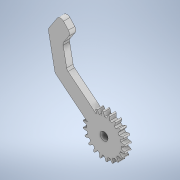
# Autodesk Inventor part: Servo pinza 1
Saved by Autodesk Inventor 2021 (Build 250183000, 183)
## iProperties
Created: 2021-03-25
Part Number: Servo pinza 1
Material: Generic
Document SubType Name: Modeling
Designer: LCG
Density: 1 g/cm^3
Appearance: Default
Author: LCG
Autodesk Inventor part; units mm, degrees
ref_plane "YZ Plane" through (0, 0, 0) normal (1, 0, 0) x (0, 1, 0)
ref_plane "XZ Plane" through (0, 0, 0) normal (0, 1, 0) x (-1, 0, 0)
ref_plane "XY Plane" through (0, 0, 0) normal (0, 0, 1) x (1, 0, 0)
sketch "Sketch1" plane through (0, 0, 0) normal (0, 0, 1) x (1, 0, 0)
  circle A0 centre (0, 0) radius 2.5
  line L0 (0, 0) -> (-15.5714, 12.5511)
  line L1 (0, 0) -> (20, 0) construction
  line L2 (-15.5714, 12.5511) -> (-18.3421, 9.1137)
  line L3 (0, 0) -> (-10.3273, 2.6535)
  line L4 (0, 0) -> (22.7557, 0) construction
  line L5 (0, 0) -> (-10.6628, 0)
  line L6 (-4.786, 9.5283) -> (-22.3661, 23.6985)
  line L7 (-22.3661, 23.6985) -> (-20.7973, 25.6449)
  circle A1 centre (-20.7973, 25.6449) radius 2.5
  line L8 (-18.3421, 9.1137) -> (-10.3273, 2.6535)
  line L9 (-23.2502, 25.1624) -> (-25.4393, 36.2891)
  line L10 (-23.2502, 25.1624) -> (-11.9102, 25.1624) construction
  line L11 (-25.4393, 36.2891) -> (-22.9863, 36.7717)
  circle A2 centre (-22.9863, 36.7717) radius 2.5
  line L12 (-25.0727, 38.149) -> (-21.9049, 42.9477)
  line L13 (-25.0727, 38.149) -> (-19.3227, 38.149) construction
  line L14 (-21.9049, 42.9477) -> (-23.9913, 44.325)
  circle A3 centre (-23.9913, 44.325) radius 2.5
  line L15 (0, 0) -> (60, 0) construction
  line L16 (-25.2189, 49.3225) -> (-22.1589, 46.0257)
  line L17 (-23.9913, 39.7871) -> (-31.8111, 44.9492)
  line L18 (-31.8111, 44.9492) -> (-29.1376, 48.9991)
  line L19 (-31.8111, 44.9492) -> (-34.1674, 41.3798)
  line L20 (-24.1412, 29.6912) -> (-32.2851, 28.089)
  line L21 (-32.2851, 28.089) -> (-34.534, 39.5199)
  line L22 (-32.2851, 28.089) -> (-30.6518, 19.787)
  line L23 (-18.3421, 9.1137) -> (-29.7677, 18.3232)
  line L24 (-18.3421, 20.455) -> (-23.8834, 13.5802)
  arc A4 (-12.5406, 2.5003) -> (-12.6967, 1.5208) centre (-12.5054, 1.9925) ccw
  line L25 (-10.3273, 2.6535) -> (-12.5406, 2.5003)
  line L26 (-10.6406, 0.6873) -> (-12.6967, 1.5208)
  line L27 (-10.6455, -0.6061) -> (-12.7079, -1.4239)
  line L28 (-10.3473, -2.5746) -> (-12.5593, -2.4045)
  arc A5 (-12.7079, -1.4239) -> (-12.5593, -2.4045) centre (-12.5203, -1.897) ccw
  line L29 (-9.9594, -3.8085) -> (-11.6763, -5.2137)
  line L30 (-9.0777, -5.5937) -> (-11.2371, -6.103)
  arc A6 (-11.6763, -5.2137) -> (-11.2371, -6.103) centre (-11.3539, -5.6076) ccw
  line L31 (-8.3337, -6.6517) -> (-9.5431, -8.5116)
  line L32 (-6.9518, -8.085) -> (-8.8547, -9.2257)
  arc A7 (-9.5431, -8.5116) -> (-8.8547, -9.2257) centre (-9.1164, -8.7891) ccw
  line L33 (-5.9217, -8.8672) -> (-6.5096, -11.0065)
  line L34 (-4.17, -9.8136) -> (-5.6369, -11.478)
  arc A8 (-6.5096, -11.0065) -> (-5.6369, -11.478) centre (-6.0188, -11.1414) ccw
  line L35 (-2.951, -10.2463) -> (-2.8619, -12.4631)
  line L36 (-0.9947, -10.6163) -> (-1.8873, -12.6474)
  arc A9 (-2.8619, -12.4631) -> (-1.8873, -12.6474) centre (-2.3533, -12.4426) ccw
  line L37 (0.298, -10.6586) -> (1.0558, -12.7438)
  line L38 (2.2743, -10.4174) -> (2.0403, -12.6236)
  arc A10 (1.0558, -12.7438) -> (2.0403, -12.6236) centre (1.5342, -12.5699) ccw
  line L39 (3.5189, -10.0654) -> (4.8738, -11.8222)
  line L40 (5.3288, -9.2357) -> (5.7755, -11.4089)
  arc A11 (4.8738, -11.8222) -> (5.7755, -11.4089) centre (5.2769, -11.5113) ccw
  line L41 (6.4079, -8.5225) -> (8.2321, -9.7852)
  line L42 (7.8806, -7.1827) -> (8.9658, -9.1178)
  arc A12 (8.2321, -9.7852) -> (8.9658, -9.1178) centre (8.5218, -9.3667) ccw
  line L43 (8.6923, -6.1756) -> (10.8137, -6.8251)
  line L44 (9.6889, -4.452) -> (11.3102, -5.9665)
  arc A13 (10.8137, -6.8251) -> (11.3102, -5.9665) centre (10.9627, -6.3384) ccw
  line L45 (10.1566, -3.2461) -> (12.3751, -3.2211)
  line L46 (10.5831, -1.3013) -> (12.5875, -2.2522)
  arc A14 (12.3751, -3.2211) -> (12.5875, -2.2522) centre (12.3693, -2.7121) ccw
  line L47 (10.6628, -0.0103) -> (12.769, 0.6868)
  line L48 (10.4788, 1.9721) -> (12.6773, 1.6744)
  arc A15 (12.769, 0.6868) -> (12.6773, 1.6744) centre (12.609, 1.17) ccw
  line L49 (10.1629, 3.2264) -> (11.9582, 4.5299)
  line L50 (9.3859, 5.0595) -> (11.5711, 5.4432)
  arc A16 (11.9582, 4.5299) -> (11.5711, 5.4432) centre (11.6591, 4.9418) ccw
  line L51 (8.7043, 6.1588) -> (10.0192, 7.9457)
  line L52 (7.4075, 7.6696) -> (9.3732, 8.6983)
  arc A17 (10.0192, 7.9457) -> (9.3732, 8.6983) centre (9.6092, 8.2474) ccw
  line L53 (6.4244, 8.5101) -> (7.135, 10.6118)
  line L54 (4.7303, 9.5561) -> (6.291, 11.1329)
  arc A18 (7.135, 10.6118) -> (6.291, 11.1329) centre (6.6528, 10.7748) ccw
  line L55 (3.5385, 10.0585) -> (3.5776, 12.2768)
  line L56 (1.6068, 10.541) -> (2.6153, 12.5171)
  arc A19 (3.5776, 12.2768) -> (2.6153, 12.5171) centre (3.0687, 12.2857) ccw
  line L57 (0.3187, 10.658) -> (-0.3173, 12.7835)
  line L58 (-1.6683, 10.5314) -> (-1.3071, 12.7204)
  arc A20 (-0.3173, 12.7835) -> (-1.3071, 12.7204) centre (-0.8049, 12.6376) ccw
  line L59 (-2.9312, 10.252) -> (-4.1823, 12.0842)
  line L60 (-4.786, 9.5283) -> (-5.1063, 11.7237)
  arc A21 (-4.1823, 12.0842) -> (-5.1063, 11.7237) centre (-4.6026, 11.7971) ccw
  arc A22 (-1.6683, 10.5314) -> (-2.9312, 10.252) centre (0, 0) ccw
  arc A23 (1.6068, 10.541) -> (0.3187, 10.658) centre (0, 0) ccw
  arc A24 (4.7303, 9.5561) -> (3.5385, 10.0585) centre (0, 0) ccw
  arc A25 (7.4075, 7.6696) -> (6.4244, 8.5101) centre (0, 0) ccw
  arc A26 (9.3859, 5.0595) -> (8.7043, 6.1588) centre (0, 0) ccw
  arc A27 (10.4788, 1.9721) -> (10.1629, 3.2264) centre (0, 0) ccw
  arc A28 (10.5831, -1.3013) -> (10.6628, 0) centre (0, 0) ccw
  arc A29 (9.6889, -4.452) -> (10.1566, -3.2461) centre (0, 0) ccw
  arc A30 (7.8806, -7.1827) -> (8.6923, -6.1756) centre (0, 0) ccw
  arc A31 (5.3288, -9.2357) -> (6.4079, -8.5225) centre (0, 0) ccw
  arc A32 (2.2743, -10.4174) -> (3.5189, -10.0654) centre (0, 0) ccw
  arc A33 (-0.9947, -10.6163) -> (0.298, -10.6586) centre (0, 0) ccw
  arc A34 (-4.17, -9.8136) -> (-2.951, -10.2463) centre (0, 0) ccw
  arc A35 (-6.9518, -8.085) -> (-5.9217, -8.8672) centre (0, 0) ccw
  arc A36 (-9.0777, -5.5937) -> (-8.3337, -6.6517) centre (0, 0) ccw
  arc A37 (-10.3473, -2.5746) -> (-9.9594, -3.8085) centre (0, 0) ccw
  arc A38 (-10.2331, 2.9964) -> (-10.3273, 2.6535) centre (0, 0) ccw
  arc A39 (-10.6406, 0.6873) -> (-10.6455, -0.6061) centre (0, 0) ccw
  line L61 (-4.9971, 9.2664) -> (-4.786, 9.5283)
  arc A40 (-25.2189, 49.3225) -> (-29.1376, 48.9991) centre (-27.0512, 47.6218) ccw
  arc A41 (-34.1674, 41.3798) -> (-34.534, 39.5199) centre (-32.081, 40.0025) ccw
  arc A42 (-30.6518, 19.787) -> (-29.7677, 18.3232) centre (-28.1988, 20.2696) ccw
  point P0 (-4.786, 9.5283)
  dimension "d0" = 5
  dimension "d1" = 20
  dimension "d2" = 141.13
  dimension "d3" = 4.415
  dimension "d4" = 165.59
  dimension "d5" = 22.58
  dimension "d6" = 2.5
  dimension "d10" = 11.34
  dimension "d12" = 101.13
  dimension "d13" = 2.5
  dimension "d15" = 5.75
  dimension "d17" = 56.57
  dimension "d18" = 2.5
  dimension "d22" = 9.37
  dimension "d23" = 8.3
  dimension "d24" = 8.83
  dimension "d25" = 1.991
  dimension "d27" = 1.018
  dimension "d30" = 300.366
  dimension "d32" = 2.5
  constraints: 124 end point, 85 point on circle, 43 centre point, 23 point on line, 15 perpendicular, 11 tangent, 6 horizontal, 5 coincident, 3 equal length, 2 equal radius, 137 other
  measures "d0" diameter of A0
  measures "d1" distance of L0.start L0.end
  measures "d2" angle of L1 L0
  measures "d3" distance of L0.end L2.end
  measures "d4" angle of L4 L3
  measures "d5" distance of L6.start L6.end
  measures "d6" distance of L6.end L7.end
  measures "d10" distance of L9.start L9.end
  measures "d12" angle of L10 L9
  measures "d13" distance of L9.end L11.end
  measures "d15" distance of L12.start L12.end
  measures "d17" angle of L13 L12
  measures "d18" distance of L12.end L14.end
  measures "d22" distance of L17.start L17.end
  measures "d23" distance of L20.start L20.end
  measures "d24" distance of L24.start L24.end
  measures "d25" distance of L3.end L26.start
  measures "d27" diameter of A4
  measures "d32" radius of A40
extrude "Extrusion1" add sketch "Sketch1" along normal blind 4 contours A0 L0 L2 L23 L24 L6 L60 A21 L59 A22 L58 A20 L57 A23 L56 A19 L55 A24 L54 A18 L53 A25 L52 A17 L51 A26 L50 A16 L49 A27 L48 A15 L47 A28 L46 A14 L45 A29 L44 A13 L43 A30 L42 A12 L41 A31 L40 A11 L39 A32 L38 A10 L37 A33 L36 A9 L35 A34 L34 A8 L33 A35 L32 A7 L31 A36 L30 A6 L29 A37 L28 A5 L27 A39 L5 | A0 L3 L8 L2 L0 | L5 A39 L26 A4 L25 L3 A0 | L23 A42 L22 L20 L9 A1 L6 L24 | L21 A41 L19 L17 L12 A2 L9 L20 | L18 A40 L16 A3 L12 L17 | A3
body "Solid1"
